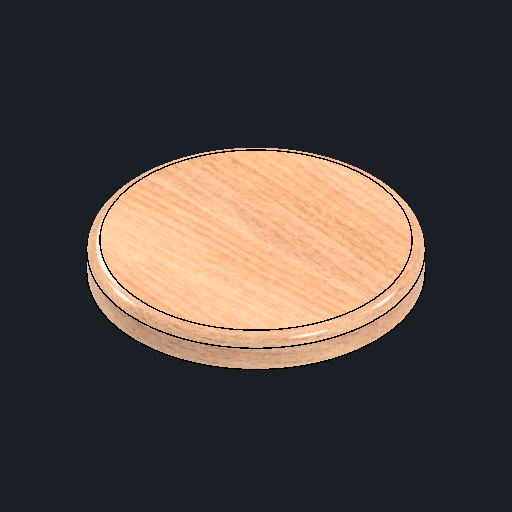
# Autodesk Inventor part: Seat
Saved by Autodesk Inventor 2026.2 (Build 302298000, 298)
## iProperties
Created: 2026-10-01
Part Number: Seat
Material: Wood (Birch)
Document SubType Name: Modeling
Designer: Joshua Eah
Density: 0.55 g/cm^3
Appearance: Birch - Natural Polished
Mass: 2058.08 g
Surface Area: 2377.52 cm^2
Volume: 3741.95 cm^3
Author: Joshua Eah
Autodesk Inventor part; units mm, degrees
ref_plane "YZ Plane" through (0, 0, 0) normal (1, 0, 0) x (0, 1, 0)
ref_plane "XZ Plane" through (0, 0, 0) normal (0, 1, 0) x (-1, 0, 0)
ref_plane "XY Plane" through (0, 0, 0) normal (0, 0, 1) x (1, 0, 0)
sketch "Sketch1" plane through (0, 0, 0) normal (0, 1, 0) x (-1, 0, 0)
  circle A0 centre (0, 0) radius 165.1
  point P0 (0, 76.2)
  point P1 (0, 101.6)
  dimension "d0" = 330.2
  dimension "d4" = 25.4
  dimension "d5" = 76.2
  constraints: 2 vertical alignment, 1 centre point, 1 coincident
  measures "d0" diameter of A0
  measures "d4" distance of point (0, 101.6) point (0, 76.2)
  measures "d5" distance of A0.centre point (0, 76.2)
extrude "Extrusion1" add sketch "Sketch1" along normal blind 38.1
fillet "Fillet1" radius 12.7 1 edges at (165.1, 38.1, 0)
hole "Hole1" at (0, 0, 76.2) at (0, 0, 101.6) direction (0, 1, 0) diameter 5.6134 depth 19.05 tip angle 118 clearance for "Flat Head Machine Screw (82)" size "#12" standard "Ansi Unified Screw Threads"
pattern_circular "Circular Pattern1" count 4 over 360 about axis through (0, -10, 0) along (0, 1, 0) of "Hole1"
body "Solid1"
